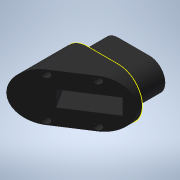
# Autodesk Inventor part: PrismSensorHolder
Saved by Autodesk Inventor 2020 (Build 240168000, 168)
## iProperties
Created: 2019-09-08
Part Number: PrismSensorHolder
Material: ABS Plastic
Document SubType Name: Modeling
Designer: vmiguel
Density: 1.06 g/cm^3
Appearance: Rubber - Black
Author: vmiguel
Autodesk Inventor part; units mm, degrees
ref_plane "YZ Plane" through (0, 0, 0) normal (1, 0, 0) x (0, 1, 0)
ref_plane "XZ Plane" through (0, 0, 0) normal (0, 1, 0) x (-1, 0, 0)
ref_plane "XY Plane" through (0, 0, 0) normal (0, 0, 1) x (1, 0, 0)
sketch "Sketch1" plane through (0, 0, 0) normal (0, 0, 1) x (1, 0, 0)
  arc A0 (-15, 23) -> (-15, -23) centre (-15, 0) ccw projected
  line L0 (15, -23) -> (-15, -23) projected
  arc A1 (15, -23) -> (15, 23) centre (15, 0) ccw projected
  line L1 (-15, 23) -> (15, 23) projected
  arc A2 (-15, 15) -> (-15, -15) centre (-15, 0) ccw projected
  line L2 (15, 15) -> (-15, 15) projected
  arc A3 (15, -15) -> (15, 15) centre (15, 0) ccw projected
  line L3 (-15, -15) -> (15, -15) projected
  point P0 (0, 0)
extrude "Extrusion1" add sketch "Sketch1" against normal blind 30 contours L2 A3 L3 A2
extrude "Extrusion2" add sketch "Sketch1" along normal blind 70 contours L1 A1 L0 A0 | L2 A3 L3 A2
sketch "Sketch2" plane through (-15, 23, 0) normal (0, 1, 0) x (1, 0, 0)
  line L0 (42.6521, -11.2963) -> (7.7634, -33.9533) projected
  line L1 (-15.3121, -126.1338) -> (136.2489, -27.709)
  line L2 (136.2489, -27.709) -> (100.9882, 26.5876)
  line L3 (100.9882, 26.5876) -> (-50.5727, -71.8372)
  line L4 (-50.5727, -71.8372) -> (-15.3121, -126.1338)
  line L5 (-15.3121, -126.1338) -> (100.9882, 26.5876) construction
  line L6 (136.2489, -27.709) -> (-50.5727, -71.8372) construction
  point P0 (15, 0)
  point P1 (42.8381, -49.7731)
  point P2 (25.2078, -22.6248)
  constraints: 12 end point, 4 midpoint, 2 parallel, 1 collinear, 1 perpendicular
extrude "Extrusion3" cut sketch "Sketch2" along normal mid plane 100
sketch "Sketch3" plane through (-15, 23, 38.9949) normal (0.544639, 0, 0.8386706) x (0.8386706, 0, -0.544639)
  arc A0 (9.2568, -24.5) -> (9.2568, -21.5) centre (9.2568, -23) ccw projected
  line L0 (9.2568, -24.5) -> (9.2568, -27.825) projected
  line L1 (9.2568, -27.825) -> (50.8568, -27.825) projected
  line L2 (50.8568, -27.825) -> (50.8568, -18.175) projected
  line L3 (50.8568, -18.175) -> (9.2568, -18.175) projected
  line L4 (9.2568, -18.175) -> (9.2568, -21.5) projected
  line L5 (7.0568, -15.5) -> (53.0568, -15.5)
  line L6 (53.0568, -15.5) -> (53.0568, -30.5)
  line L7 (53.0568, -30.5) -> (7.0568, -30.5)
  line L8 (7.0568, -30.5) -> (7.0568, -15.5)
  line L9 (7.0568, -15.5) -> (53.0568, -30.5) construction
  line L10 (53.0568, -15.5) -> (7.0568, -30.5) construction
  point P0 (33.8182, -23)
  point P1 (30.0568, -23)
  dimension "d6" = 46
  dimension "d7" = 15
  constraints: 12 end point, 2 midpoint, 2 parallel, 1 horizontal, 1 perpendicular
  measures "d6" distance of L6.end L7.end
  measures "d7" distance of L5.end L6.end
extrude "Extrusion4" cut sketch "Sketch3" against normal blind 35 contours A0 L4 L3 L2 L1 L0 | L5 L6 L7 L8
sketch "Sketch5" plane through (0, 0, 0) normal (0, 1, 0) x (-1, 0, 0)
  line L0 (-18.6362, 8.5425) -> (-4.6475, -28.9317) projected
  line L1 (-4.6475, -28.9317) -> (20.8118, 1.9199) projected
  line L2 (20.5595, 1.9623) -> (-18.6362, 8.5425) projected
  line L3 (20.5258, 1.4948) -> (-4.2075, -28.4771)
  line L4 (-4.8761, -28.6053) -> (-18.595, 8.1461)
  line L5 (-18.2398, 8.5773) -> (20.317, 2.054)
  arc A0 (-4.8446, -28.7851) -> (-4.3218, -28.7903) centre (-4.5832, -28.7877) ccw
  arc A1 (-4.8446, -28.7851) -> (-4.8761, -28.6053) centre (-5.3446, -28.7801) ccw
  arc A2 (-4.2075, -28.4771) -> (-4.3218, -28.7903) centre (-3.8218, -28.7953) ccw
  arc A3 (-18.5791, 8.8033) -> (-18.8814, 8.4369) centre (-18.7905, 8.6698) ccw
  arc A4 (-18.595, 8.1461) -> (-18.8814, 8.4369) centre (-19.0634, 7.9712) ccw
  arc A5 (-18.5791, 8.8033) -> (-18.2398, 8.5773) centre (-18.1564, 9.0703) ccw
  line L6 (-4.6475, -28.9317) -> (20.8118, 1.9199) projected
  line L7 (20.5595, 1.9623) -> (-18.6362, 8.5425) projected
  arc A6 (20.845, 1.6721) -> (20.6746, 2.129) centre (20.8118, 1.9199) ccw
  arc A7 (20.845, 1.6721) -> (20.5258, 1.4948) centre (20.9114, 1.1766) ccw
  arc A8 (20.317, 2.054) -> (20.6746, 2.129) centre (20.4004, 2.547) ccw
  point P0 (0, 0)
  point P1 (-4.3565, -28.6576)
  point P2 (-18.5438, 8.6288)
  point P3 (-4.8347, -28.7163)
  point P4 (-18.703, 8.4356)
  point P5 (20.5785, 2.0098)
  point P6 (20.6944, 1.6992)
  dimension "d10" = 0.1
  dimension "d12" = 0.5
  dimension "d13" = 0.5
  dimension "d14" = 0.5
  dimension "d15" = 0.5
  dimension "d16" = 0.5
  constraints: 24 point on circle, 12 tangent, 9 centre point, 6 end point, 6 point on line, 3 equal radius, 1 coincident
  measures "d10" distance between parallel lines of L0 L4
  measures "d12" radius of A1
  measures "d13" diameter of A3
  measures "d14" radius of A4
  measures "d15" diameter of A6
  measures "d16" radius of A7
extrude "Extrusion5" cut sketch "Sketch5" along normal mid plane 20.1
sketch "Sketch6" plane through (0, 0, -30) normal (0, 0, -1) x (-1, 0, 0)
  arc A0 (-15, 15) -> (-15, -15) centre (-15, 0) ccw projected
  line L0 (-15, -15) -> (15, -15) projected
  arc A1 (15, -15) -> (15, 15) centre (15, 0) ccw projected
  line L1 (15, 15) -> (-15, 15) projected
  arc A2 (15, -9) -> (15, 9) centre (15, 0) ccw
  line L2 (15, -9) -> (-15, -9)
  arc A3 (-15, 9) -> (-15, -9) centre (-15, 0) ccw
  line L3 (-15, 9) -> (15, 9)
  point P0 (0, 0)
  dimension "d19" = 6
  constraints: 4 end point, 4 point on circle, 2 centre point, 3 other
  measures "d19" radial gap between concentric circles of A1 A2
extrude "Extrusion6" cut sketch "Sketch6" against normal blind 40 contours L2 A3 L3 A2
split body "Split1" result two bodies by plane through (0, 0, 0) normal (0, 1, 0) first body at (-24.0717, 20.5902, 29.8229)
fillet "Fillet1" radius 8 2 edges at (-28.1451, 3.75, 5.7964) (-28.1451, -3.75, 5.7964)
ref_plane "Work Plane1" through (0, 0, 55) normal (0, 0, -1) x (-1, 0, 0)
sketch "Sketch7" plane through (0, 0, 55) normal (0, 0, -1) x (-1, 0, 0)
  line L0 (-30, 0) -> (-38, 0) projected
  arc A0 (-15, 15) -> (-30, 0) centre (-15, 0) ccw projected
  line L1 (-15, 15) -> (15, 15) projected
  arc A1 (30, 0) -> (15, 15) centre (15, 0) ccw projected
  line L2 (38, 0) -> (30, 0) projected
  arc A2 (38, 0) -> (15, 23) centre (15, 0) ccw projected
  line L3 (-15, 23) -> (15, 23) projected
  arc A3 (-15, 23) -> (-38, 0) centre (-15, 0) ccw projected
  line L4 (-30, 0) -> (-38, 0) projected
  arc A4 (-38, 0) -> (-15, -23) centre (-15, 0) ccw projected
  line L5 (15, -23) -> (-15, -23) projected
  arc A5 (15, -23) -> (38, 0) centre (15, 0) ccw projected
  line L6 (38, 0) -> (30, 0) projected
  arc A6 (15, -15) -> (30, 0) centre (15, 0) ccw projected
  line L7 (15, -15) -> (-15, -15) projected
  arc A7 (-30, 0) -> (-15, -15) centre (-15, 0) ccw projected
  arc A8 (-15, 15) -> (-30, 0) centre (-15, 0) ccw projected
  arc A9 (-15, 23) -> (-38, 0) centre (-15, 0) ccw projected
  line L8 (-15, 15) -> (-15, 23)
  line L9 (15, 15) -> (-15, 15) projected
  line L10 (15, 15) -> (15, 23)
  line L11 (15, -15) -> (-15, -15) projected
  line L12 (15, -15) -> (15, -23)
  arc A10 (-30, 0) -> (-15, -15) centre (-15, 0) ccw projected
  line L13 (-15, -15) -> (-15, -23)
  point P0 (0, 0)
  point P1 (-15, 19)
  point P2 (15, 19)
  point P3 (15, -19)
  point P4 (-15, -19)
  constraints: 8 end point, 4 midpoint, 2 perpendicular, 1 parallel, 1 vertical
hole "Hole1" at (15, 19, 55) at (-15, 19, 55) at (15, -19, 55) at (-15, -19, 55) direction (0, 0, -1) diameter 3 end through all counterbore diameter 6 counterbore depth 50 bodies 2 3
body "Solid2"
body "Solid3"
